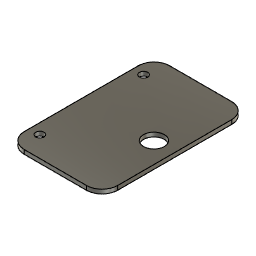
piston plate (Autodesk Fusion 360 design; units mm, degrees)
Autodesk Fusion 360 part; units mm, degrees
note: some values were not read from the file. Set by a fixed rule: which sketch regions a step uses.
sketch "Esquisse1" plane through (0, 0, 0) normal (0, 0, 1) x (1, 0, 0)
  line L0 (22.5, 35) -> (-22.5, 35)
  line L1 (-22.5, 35) -> (-22.5, -35)
  line L2 (-22.5, -35) -> (22.5, -35)
  line L3 (22.5, -35) -> (22.5, 35)
  line L4 (22.5, 35) -> (-22.5, -35) construction
  line L5 (-22.5, 35) -> (22.5, -35) construction
  dimension "d1" = 45
  dimension "d2" = 70
  constraint horizontal L0
  constraint perpendicular L0 L1
  constraint parallel L0 L2
  constraint parallel L1 L3
  constraint coincident L4 origin
  constraint coincident L5 origin
  measures "d1" distance of L1.end L2.end
  measures "d2" distance of L0.end L1.end
extrude "Face1" add sketch "Esquisse1" along normal blind 2
sketch "Esquisse2" plane through (0, 0, 2) normal (0, 0, 1) x (-1, 0, 0)
  line L0 (-22.5, 35) -> (-22.5, -35)
  line L1 (-22.5, -35) -> (22.5, -35)
  line L2 (22.5, -35) -> (22.5, 35)
  line L3 (22.5, 35) -> (-22.5, 35)
  circle A0 centre (17.5, -25) radius 2
  line L4 (-1.75, 0) -> (-22.5, 0)
  circle A1 centre (17.5, 25) radius 2
  circle A2 centre (-12.5, 0) radius 5
  dimension "d4" = 5
  dimension "d5" = 4
  dimension "d6" = 10
  dimension "d7" = 10
  dimension "d8" = 10
  constraint symmetric A0 L4 A1
  constraint coincident L4 A2.centre
  measures "d4" distance of L2 A0.centre
  measures "d5" diameter of A0
  measures "d6" distance of L1 A0.centre
  measures "d7" diameter of A2
  measures "d8" distance of L0 A2.centre
extrude "Extrusion1" cut sketch "Esquisse2" against normal through all contours A0 | L4 A2 | L4 A2 | A1
fillet "Congé1" radius 7.5 4 edges at (-22.5, -35, 1) (22.5, -35, 1) (22.5, 35, 1) (-22.5, 35, 1)
